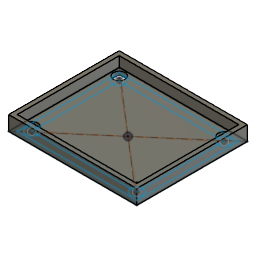
EnclosureAbove (Autodesk Fusion 360 design; units mm, degrees)
part number: 2026-09-07-19-56-31-620
Autodesk Fusion 360 part; units mm, degrees
note: some values were not read from the file. Set by a fixed rule: which sketch regions a step uses.
sketch "Sketch1" plane through (0, 0, 0) normal (0, 1, 0) x (1, 0, 0)
  line L0 (-41, -35) -> (-41, 35)
  line L1 (41, -35) -> (-41, 35) construction
  line L2 (36, -30) -> (-36, -30)
  circle A0 centre (36, -30) radius 4
  circle A1 centre (-36, -30) radius 4
  line L3 (41, -35) -> (-41, -35)
  circle A2 centre (-36, 30) radius 4
  line L4 (-41, -35) -> (41, 35) construction
  line L5 (36, -30) -> (-36, 30) construction
  circle A3 centre (36, 30) radius 4
  line L6 (-36, -30) -> (36, 30) construction
  line L7 (36, 30) -> (36, -30)
  line L8 (-41, 35) -> (41, 35)
  line L9 (41, 35) -> (41, -35)
  line L10 (-36, 30) -> (36, 30)
  line L11 (-36, -30) -> (-36, 30)
  line L12 (44, 38) -> (-44, 38)
  line L13 (-44, 38) -> (-44, -38)
  line L14 (-44, -38) -> (44, -38)
  line L15 (44, -38) -> (44, 38)
  line L16 (44, 38) -> (-44, -38) construction
  line L17 (-44, 38) -> (44, -38) construction
  dimension "d1" = 82
  dimension "d2" = 70
  dimension "d3" = 60
  dimension "d4" = 72
  dimension "d5" = 8
  dimension "d6" = 8
  dimension "d7" = 8
  dimension "d8" = 8
  dimension "d9" = 88
  dimension "d10" = 76
  constraint horizontal L3
  constraint perpendicular L0 L3
  constraint parallel L3 L8
  constraint parallel L0 L9
  constraint horizontal L2
  constraint perpendicular L2 L11
  constraint parallel L2 L10
  constraint parallel L7 L11
  constraint coincident A2.centre L5.end
  constraint coincident A3.centre L6.end
  constraint coincident L2.end A1.centre
  constraint coincident L2.start A0.centre
  constraint horizontal L12
  constraint perpendicular L12 L13
  constraint parallel L12 L14
  constraint parallel L13 L15
  constraint coincident L16 origin
  constraint coincident L17 origin
  measures "d1" distance of L4.end L0.end
  measures "d2" distance of L1.start L4.end
  measures "d3" distance of A3.centre L2.start
  measures "d4" distance of A3.centre A2.centre
  measures "d5" diameter of A2
  measures "d6" diameter of A3
  measures "d7" diameter of A1
  measures "d8" diameter of A0
  measures "d9" distance of L13.end L14.end
  measures "d10" distance of L12.end L13.end
extrude "Extrude1" add sketch "Sketch1" along normal blind 3 contours L0 L3 L8 L9 makes body 1
extrude "Extrude2" add sketch "Sketch1" along normal blind 10 separate body contours L12 L13 L14 L15 makes body 2
extrude "Extrude3" add sketch "Sketch1" along normal blind 3 contours L2 A1 L11 | L2 A0 A1 A2 A3 L7 L10 L11 | L2 A1 L11 | L2 A0 L7 | L2 A0 L7 | A2 L10 L11 | A2 L10 L11 | A3 L7 L10 | A3 L7 L10 bodies 1
extrude "Extrude4" cut sketch "Sketch1" along normal blind 10 contours L2 A1 L11 | L2 A1 L11 | L2 A0 L7 | L2 A0 L7 | A2 L10 L11 | A2 L10 L11 | A3 L7 L10 | A3 L7 L10 bodies 1
